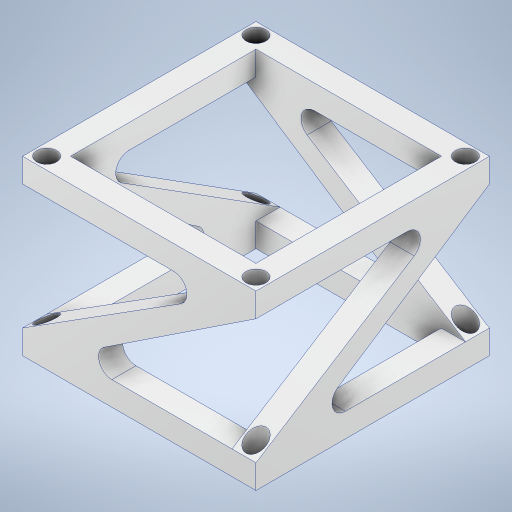
# Autodesk Inventor part: SolarCar
Saved by Autodesk Inventor 2024 (Build 280153000, 153)
## iProperties
Created: 2024-09-23
Part Number: SolarCar
Material: Aluminum 6061
Document SubType Name: Modeling
Designer: furqa
Density: 2.7 g/cm^3
Appearance: Aluminum - Flat
Mass: 13.1533 g
Surface Area: 54.7388 cm^2
Volume: 4.8716 cm^3
Author: furqa
Autodesk Inventor part; units mm, degrees
ref_plane "YZ Plane" through (0, 0, 0) normal (1, 0, 0) x (0, 1, 0)
ref_plane "XZ Plane" through (0, 0, 0) normal (0, 1, 0) x (-1, 0, 0)
ref_plane "XY Plane" through (0, 0, 0) normal (0, 0, 1) x (1, 0, 0)
sketch "Sketch1" plane through (0, 0, 0) normal (0, 1, 0) x (-1, 0, 0)
  line L0 (0, 0) -> (35, 0)
  line L1 (35, 0) -> (35, 35)
  line L2 (35, 35) -> (0, 35)
  line L3 (0, 35) -> (0, 0)
  line L4 (3.6, 3.6) -> (31.4, 3.6)
  line L5 (31.4, 3.6) -> (31.4, 31.4)
  line L6 (31.4, 31.4) -> (3.6, 31.4)
  line L7 (3.6, 31.4) -> (3.6, 3.6)
  circle A0 centre (33.2, 33.2) radius 1.5
  circle A1 centre (33.2, 1.8) radius 1.5
  circle A2 centre (1.8, 1.8) radius 1.5
  circle A3 centre (1.8, 33.2) radius 1.5
  dimension "d0" = 35
  dimension "d1" = 35
  dimension "d2" = 3.6
  dimension "d3" = 3.6
  dimension "d4" = 3.6
  dimension "d5" = 3.6
  dimension "d6" = 3
  dimension "d7" = 1.8
  dimension "d8" = 1.8
  dimension "d9" = 3
  dimension "d10" = 1.8
  dimension "d11" = 1.8
  dimension "d12" = 3
  dimension "d13" = 1.8
  dimension "d14" = 1.8
  dimension "d15" = 3
  dimension "d16" = 1.8
  dimension "d17" = 1.8
  constraints: 16 end point, 4 centre point, 4 parallel, 2 horizontal, 2 perpendicular
  measures "d0" distance of L0.end L1.end
  measures "d1" distance of L1.end L2.end
  measures "d2" distance between parallel lines of L1 L5
  measures "d3" distance between parallel lines of L2 L6
  measures "d4" distance between parallel lines of L0 L4
  measures "d5" distance between parallel lines of L3 L7
  measures "d6" diameter of A0
  measures "d7" distance from line of L1 A0.centre
  measures "d8" distance from line of L2 A0.centre
  measures "d9" diameter of A1
  measures "d10" distance from line of L0 A1.centre
  measures "d11" distance from line of L1 A1.centre
  measures "d12" diameter of A2
  measures "d13" distance from line of L0 A2.centre
  measures "d14" distance from line of L3 A2.centre
  measures "d15" diameter of A3
  measures "d16" distance from line of L2 A3.centre
  measures "d17" distance from line of L3 A3.centre
extrude "Extrusion1" add sketch "Sketch1" along normal blind 25.9
sketch "Sketch3" plane through (-35, 0, 35) normal (0, 0, 1) x (1, 0, 0)
  line L0 (0, 25.9) -> (35, 25.9) projected
  line L1 (0, 0) -> (35, 0) projected
  line L2 (0, 0) -> (0, 25.9) projected
  line L3 (18.01, 21.1181) -> (18.01, 21.1181)
  line L4 (0, 0) -> (0, 25.9) projected
  line L5 (31.4, 0) -> (31.4, 25.9) projected
  line L6 (31.4, 3.6) -> (13.39, 3.6)
  arc A0 (12.1285, 7.1519) -> (13.39, 3.6) centre (13.39, 5.6) ccw
  line L7 (3.6, 22.3) -> (22.6522, 22.3)
  line L8 (3.6, 22.3) -> (0, 22.3)
  line L9 (31.4, 3.6) -> (31.4, 0)
  line L10 (0, 22.3) -> (0, 25.9)
  line L11 (31.4, 22.2467) -> (31.4, 25.9)
  line L12 (0, 3.6) -> (0, 0)
  line L13 (35, 0) -> (35, 25.9) projected
  line L14 (31.4, 20.2467) -> (31.4, 25.9)
  line L15 (0, 25.9) -> (0, 22.3)
  line L16 (12.1285, 7.1519) -> (35, 22.3)
  arc A1 (23.7216, 18.6099) -> (22.6522, 22.3) centre (22.6522, 20.3) ccw
  line L17 (0, 3.6) -> (23.7216, 18.6099)
  line L18 (3.6, 22.3) -> (3.6, 5.8779)
  line L19 (3.6, 0) -> (3.6, 25.9) projected
  line L20 (35, 12.95) -> (31.4, 12.95)
  line L21 (3.6, 5.8779) -> (3.6, 12.95)
  line L22 (0, 12.95) -> (0, 3.6)
  line L23 (0, 12.95) -> (3.6, 12.95)
  point P0 (31.4, 19.9157)
  point P1 (0, 22.3)
  dimension "d41" = 18.01
  dimension "d42" = 4
  dimension "d50" = 3.6
  dimension "d67" = 3.6
  dimension "d70" = 3.6
  dimension "d71" = 4
  constraints: 34 end point, 8 point on line, 7 collinear, 4 midpoint, 4 point on circle, 3 perpendicular, 2 centre point, 1 parallel, 1 tangent, 1 vertical
  measures "d41" distance of L6.start L6.end
  measures "d42" diameter of A0
  measures "d50" distance of L0.end L16.end
  measures "d67" distance between parallel lines of L1 L6
  measures "d70" distance between parallel lines of L7 L0
  measures "d71" diameter of A1
extrude "Extrusion2" cut sketch "Sketch3" against normal blind 3.6 contours L7 A1 L17 L18 | L23 L18 L17 L2 | L13 L20 L5 L16 | L5 L6 A0 L16
sketch "Sketch8" plane through (0, 0, 0) normal (0, 0, -1) x (-1, 0, 0)
  line L0 (0, 25.9) -> (35, 25.9)
  line L1 (0, 0) -> (35, 0)
  line L2 (0, 0) -> (0, 25.9)
  line L3 (18.01, 21.1181) -> (18.01, 21.1181)
  line L4 (0, 0) -> (0, 25.9)
  line L5 (31.4, 0) -> (31.4, 25.9)
  line L6 (31.4, 3.6) -> (13.39, 3.6)
  arc A0 (12.1285, 7.1519) -> (13.39, 3.6) centre (13.39, 5.6) ccw
  line L7 (3.6, 22.3) -> (22.6522, 22.3)
  line L8 (3.6, 22.3) -> (0, 22.3)
  line L9 (31.4, 3.6) -> (31.4, 0)
  line L10 (0, 22.3) -> (0, 25.9)
  line L11 (31.4, 22.2467) -> (31.4, 25.9)
  line L12 (0, 3.6) -> (0, 0)
  line L13 (35, 0) -> (35, 25.9)
  line L14 (31.4, 20.2467) -> (31.4, 25.9)
  line L15 (0, 25.9) -> (0, 22.3)
  line L16 (12.1285, 7.1519) -> (35, 22.3)
  arc A1 (23.7216, 18.6099) -> (22.6522, 22.3) centre (22.6522, 20.3) ccw
  line L17 (0, 3.6) -> (23.7216, 18.6099)
  line L18 (3.6, 22.3) -> (3.6, 5.8779)
  line L19 (3.6, 0) -> (3.6, 25.9)
  line L20 (35, 12.95) -> (31.4, 12.95)
  line L21 (3.6, 5.8779) -> (3.6, 12.95)
  line L22 (0, 12.95) -> (0, 3.6)
  line L23 (0, 12.95) -> (3.6, 12.95)
  point P0 (31.4, 19.9157)
  point P1 (0, 22.3)
  dimension "d80" = 18.01
  dimension "d78" = 4
  dimension "d76" = 3.6
  dimension "d79" = 3.6
  dimension "d77" = 3.6
  dimension "d75" = 4
  constraints: 48 end point, 8 point on line, 7 collinear, 4 midpoint, 4 point on circle, 3 perpendicular, 2 centre point, 1 parallel, 1 tangent, 1 vertical
  measures "d80" distance of L6.start L6.end
  measures "d78" diameter of A0
  measures "d76" distance of L0.end L16.end
  measures "d79" distance between parallel lines of L1 L6
  measures "d77" distance between parallel lines of L7 L0
  measures "d75" diameter of A1
extrude "Extrusion4" cut sketch "Sketch8" against normal blind 3.6 contours L7 A1 L17 L18 | L23 L18 L17 L2 | L13 L20 L5 L16 | L5 L6 A0 L16
sketch "Sketch9" plane through (0, 0, 35) normal (1, 0, 0) x (0, 0, -1)
  line L0 (0, 25.9) -> (35, 25.9)
  line L1 (0, 0) -> (35, 0)
  line L2 (0, 0) -> (0, 25.9)
  line L3 (18.01, 21.1181) -> (18.01, 21.1181)
  line L4 (0, 0) -> (0, 25.9)
  line L5 (31.4, 0) -> (31.4, 25.9)
  line L6 (31.4, 3.6) -> (13.39, 3.6)
  arc A0 (12.1285, 7.1519) -> (13.39, 3.6) centre (13.39, 5.6) ccw
  line L7 (3.6, 22.3) -> (22.6522, 22.3)
  line L8 (3.6, 22.3) -> (0, 22.3)
  line L9 (31.4, 3.6) -> (31.4, 0)
  line L10 (0, 22.3) -> (0, 25.9)
  line L11 (31.4, 22.2467) -> (31.4, 25.9)
  line L12 (0, 3.6) -> (0, 0)
  line L13 (35, 0) -> (35, 25.9)
  line L14 (31.4, 20.2467) -> (31.4, 25.9)
  line L15 (0, 25.9) -> (0, 22.3)
  line L16 (12.1285, 7.1519) -> (35, 22.3)
  arc A1 (23.7216, 18.6099) -> (22.6522, 22.3) centre (22.6522, 20.3) ccw
  line L17 (0, 3.6) -> (23.7216, 18.6099)
  line L18 (3.6, 22.3) -> (3.6, 5.8779)
  line L19 (3.6, 0) -> (3.6, 25.9)
  line L20 (35, 12.95) -> (31.4, 12.95)
  line L21 (3.6, 5.8779) -> (3.6, 12.95)
  line L22 (0, 12.95) -> (0, 3.6)
  line L23 (0, 12.95) -> (3.6, 12.95)
  point P0 (31.4, 19.9157)
  point P1 (0, 22.3)
  dimension "d89" = 18.01
  dimension "d87" = 4
  dimension "d85" = 3.6
  dimension "d88" = 3.6
  dimension "d86" = 3.6
  dimension "d84" = 4
  constraints: 48 end point, 8 point on line, 7 collinear, 4 midpoint, 4 point on circle, 3 perpendicular, 2 centre point, 1 parallel, 1 tangent, 1 vertical
  measures "d89" distance of L6.start L6.end
  measures "d87" diameter of A0
  measures "d85" distance of L0.end L16.end
  measures "d88" distance between parallel lines of L1 L6
  measures "d86" distance between parallel lines of L7 L0
  measures "d84" diameter of A1
extrude "Extrusion5" cut sketch "Sketch9" against normal blind 3.6 contours L7 A1 L17 L18 | L23 L18 L17 L2 | L13 L20 L5 L16 | L5 L6 A0 L16
sketch "Sketch10" plane through (-35, 0, 0) normal (-1, 0, 0) x (0, 0, 1)
  line L0 (0, 25.9) -> (35, 25.9)
  line L1 (0, 0) -> (35, 0)
  line L2 (0, 0) -> (0, 25.9)
  line L3 (18.01, 21.1181) -> (18.01, 21.1181)
  line L4 (0, 0) -> (0, 25.9)
  line L5 (31.4, 0) -> (31.4, 25.9)
  line L6 (31.4, 3.6) -> (13.39, 3.6)
  arc A0 (12.1285, 7.1519) -> (13.39, 3.6) centre (13.39, 5.6) ccw
  line L7 (3.6, 22.3) -> (22.6522, 22.3)
  line L8 (3.6, 22.3) -> (0, 22.3)
  line L9 (31.4, 3.6) -> (31.4, 0)
  line L10 (0, 22.3) -> (0, 25.9)
  line L11 (31.4, 22.2467) -> (31.4, 25.9)
  line L12 (0, 3.6) -> (0, 0)
  line L13 (35, 0) -> (35, 25.9)
  line L14 (31.4, 20.2467) -> (31.4, 25.9)
  line L15 (0, 25.9) -> (0, 22.3)
  line L16 (12.1285, 7.1519) -> (35, 22.3)
  arc A1 (23.7216, 18.6099) -> (22.6522, 22.3) centre (22.6522, 20.3) ccw
  line L17 (0, 3.6) -> (23.7216, 18.6099)
  line L18 (3.6, 22.3) -> (3.6, 5.8779)
  line L19 (3.6, 0) -> (3.6, 25.9)
  line L20 (35, 12.95) -> (31.4, 12.95)
  line L21 (3.6, 5.8779) -> (3.6, 12.95)
  line L22 (0, 12.95) -> (0, 3.6)
  line L23 (0, 12.95) -> (3.6, 12.95)
  point P0 (31.4, 19.9157)
  point P1 (0, 22.3)
  dimension "d98" = 18.01
  dimension "d96" = 4
  dimension "d94" = 3.6
  dimension "d97" = 3.6
  dimension "d95" = 3.6
  dimension "d93" = 4
  constraints: 48 end point, 8 point on line, 7 collinear, 4 midpoint, 4 point on circle, 3 perpendicular, 2 centre point, 1 parallel, 1 tangent, 1 vertical
  measures "d98" distance of L6.start L6.end
  measures "d96" diameter of A0
  measures "d94" distance of L0.end L16.end
  measures "d97" distance between parallel lines of L1 L6
  measures "d95" distance between parallel lines of L7 L0
  measures "d93" diameter of A1
extrude "Extrusion6" cut sketch "Sketch10" against normal blind 3.6 contours L7 A1 L17 L18 | L23 L18 L17 L2 | L13 L20 L5 L16 | L5 L6 A0 L16
body "Solid1"
